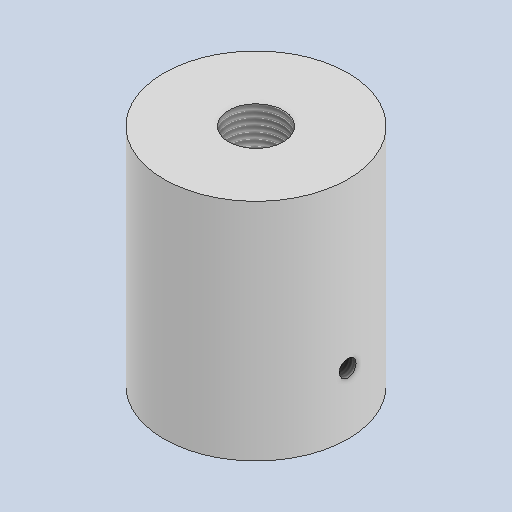
# Autodesk Inventor part: 17701729.304517.015
Saved by Autodesk Inventor 2023 (Build 270158000, 158)
## iProperties
Created: 2022-05-01
Part Number: 17701729.304517.015
Material: Типовые
Document SubType Name: Modeling
Designer: User
Density: 1 g/cm^3
Appearance: По умолчанию
Author: User
Title: Маховик
Autodesk Inventor part; units mm, degrees
ref_plane "YZ Plane" through (0, 0, 0) normal (1, 0, 0) x (0, 1, 0)
ref_plane "XZ Plane" through (0, 0, 0) normal (0, 1, 0) x (-1, 0, 0)
sketch "Эскиз1" plane through (0, 0, 0) normal (0, 1, 0) x (-1, 0, 0)
  circle A0 centre (0, 0) radius 22.5
  dimension "d0" = 45
  constraints: 1 centre point, 1 coincident
  measures "d0" diameter of A0
extrude "Выдавливание1" add sketch "Эскиз1" along normal blind 55
sketch "Эскиз2" plane through (0, 0, 0) normal (0, -1, 0) x (1, 0, 0)
  circle A0 centre (0, 0) radius 22.5 projected
  point P0 (22.5, 0)
  constraints: 1 horizontal alignment, 1 other
ref_plane "РабПлоскость1" through (22.5, 0, 0) normal (1, 0, 0) x (0, 1, 0)
sketch "Эскиз3" plane through (22.5, 0, 0) normal (1, 0, 0) x (0, 1, 0)
  line L0 (0, 0) -> (12.5, 0)
  line L1 (12.5, 0) -> (17.5, 0)
  circle A0 centre (15, 0) radius 2.5
  dimension "d3" = 12.5
  dimension "d4" = 5
  constraints: 4 end point, 1 horizontal, 1 horizontal alignment, 1 midpoint, 1 point on line, 2 other
  measures "d3" distance of L0.start L0.end
  measures "d4" distance of L0.end L1.end
hole "Отверстие1" at (22.5, 15, 0) direction (-1, 0, 0) diameter 4.134 depth 10 tip angle 118 thread size "M5x0.8" class "6H" standard "ISO Metric profile"
sketch "Эскиз4" plane through (0, 55, 0) normal (0, 1, 0) x (1, 0, 0)
  point P0 (0, 0)
  point P1 (0, 0)
  constraints: 1 coincident
hole "Отверстие2" at (0, 55, 0) direction (0, -1, 0) diameter 13.3762 depth 20 thread size "M15x1.5" class "6H" standard "ISO Metric profile"
sketch "Эскиз5" plane through (0, 0, 0) normal (0, -1, 0) x (1, 0, 0)
  circle A0 centre (0, 0) radius 8
  dimension "d27" = 16
  constraints: 1 centre point, 1 coincident
  measures "d27" diameter of A0
extrude "Выдавливание2" cut sketch "Эскиз5" against normal blind 4
